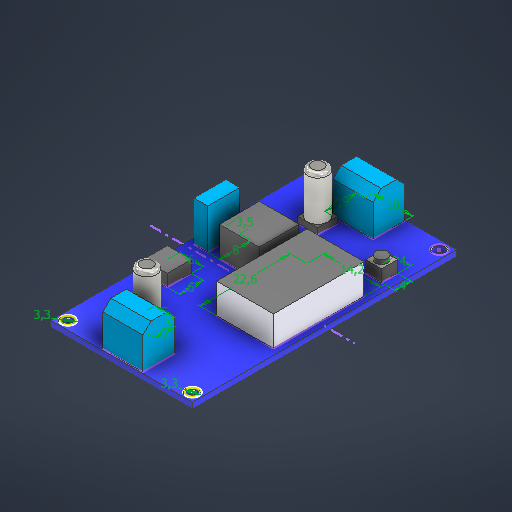
# Autodesk Inventor part: STEP_DOWN_LM2596
Saved by Autodesk Inventor 2027.1 (Build 311270010, 270A)
## iProperties
Created: 2026-08-16
Part Number: STEP_DOWN_LM2596
Material: Genérico
Document SubType Name: Modeling
Designer: Evellyn
Density: 1 g/cm^3
Appearance: Padrão
Author: Evellyn
Autodesk Inventor part; units mm, degrees
ref_plane "YZ Plane" through (0, 0, 0) normal (1, 0, 0) x (0, 1, 0)
ref_plane "XZ Plane" through (0, 0, 0) normal (0, 1, 0) x (-1, 0, 0)
ref_plane "XY Plane" through (0, 0, 0) normal (0, 0, 1) x (1, 0, 0)
sketch "Esboço1" plane through (0, 0, 0) normal (0, 1, 0) x (-1, 0, 0)
  line L0 (-17.7, -33) -> (17.7, -33)
  line L1 (17.7, -33) -> (17.7, 33)
  line L2 (17.7, 33) -> (-17.7, 33)
  line L3 (-17.7, 33) -> (-17.7, -33)
  line L4 (-17.7, -33) -> (17.7, 33) construction
  line L5 (17.7, -33) -> (-17.7, 33) construction
  circle A0 centre (15.55, 30.85) radius 1.35
  circle A1 centre (-15.55, 30.85) radius 1.35
  circle A2 centre (15.55, -30.85) radius 1.35
  circle A3 centre (-15.55, -30.85) radius 1.35
  point P0 (0, 0)
  dimension "d0" = 35.4
  dimension "d1" = 66
  dimension "d2" = 2.7
  dimension "d4" = 0.8
  dimension "d5" = 0.8
  dimension "d6" = 2.7
  dimension "d8" = 0.8
  dimension "d9" = 0.8
  constraints: 12 end point, 4 centre point, 2 midpoint, 2 parallel, 1 horizontal, 1 perpendicular
  measures "d0" distance of L2.end L1.end
  measures "d1" distance of L1.end L0.end
  measures "d2" diameter of A0
  measures "d4" distance edge to line of A0 L2
  measures "d5" distance edge to line of A0 L1
  measures "d6" diameter of A1
  measures "d8" distance edge to line of A1 L3
  measures "d9" distance edge to line of A1 L2
extrude "Extrusão1" add sketch "Esboço1" along normal blind 1.5
sketch "Esboço2" plane through (0, 1.5, 0) normal (0, 1, 0) x (1, 0, 0)
  line L0 (5, 24.7918) -> (-5, 24.7918)
  line L1 (-5, 24.7918) -> (-5, 32.6918)
  line L2 (-5, 32.6918) -> (5, 32.6918)
  line L3 (5, 32.6918) -> (5, 24.7918)
  line L4 (5, 24.7918) -> (-5, 32.6918) construction
  line L5 (-5, 24.7918) -> (5, 32.6918) construction
  line L6 (-26.0305, 0) -> (25.0606, 0)
  line L7 (5, -24.7918) -> (-5, -24.7918)
  line L8 (-5, -24.7918) -> (-5, -32.6918)
  line L9 (-5, -32.6918) -> (5, -32.6918)
  line L10 (5, -32.6918) -> (5, -24.7918)
  line L11 (16.2337, -11.3) -> (2.0337, -11.3)
  line L12 (2.0337, -11.3) -> (2.0337, 11.3)
  line L13 (2.0337, 11.3) -> (16.2337, 11.3)
  line L14 (16.2337, 11.3) -> (16.2337, -11.3)
  line L15 (16.2337, -11.3) -> (2.0337, 11.3) construction
  line L16 (2.0337, -11.3) -> (16.2337, 11.3) construction
  line L17 (-7.8666, -23.8534) -> (-2.8666, -23.8534)
  line L18 (-2.8666, -23.8534) -> (-2.8666, -18.8534)
  line L19 (-2.8666, -18.8534) -> (-7.8666, -18.8534)
  line L20 (-7.8666, -18.8534) -> (-7.8666, -23.8534)
  line L21 (-7.8666, 23.8534) -> (-2.8666, 23.8534)
  line L22 (-2.8666, 23.8534) -> (-2.8666, 18.8534)
  line L23 (-2.8666, 18.8534) -> (-7.8666, 18.8534)
  line L24 (-7.8666, 18.8534) -> (-7.8666, 23.8534)
  line L25 (11.4703, 16.4532) -> (15.4703, 16.4532)
  line L26 (15.4703, 16.4532) -> (15.4703, 20.4532)
  line L27 (15.4703, 20.4532) -> (11.4703, 20.4532)
  line L28 (11.4703, 20.4532) -> (11.4703, 16.4532)
  line L29 (-16.3029, 1.3386) -> (-12.8029, 1.3386)
  line L30 (-12.8029, 1.3386) -> (-12.8029, 9.3386)
  line L31 (-12.8029, 9.3386) -> (-16.3029, 9.3386)
  line L32 (-16.3029, 9.3386) -> (-16.3029, 1.3386)
  line L33 (-9.8893, 1.3386) -> (0, 1.3386)
  line L34 (0, 1.3386) -> (0, 11.3)
  line L35 (0, 11.3) -> (-9.8893, 11.3)
  line L36 (-9.8893, 11.3) -> (-9.8893, 1.3386)
  line L37 (-16.3029, -11.3) -> (-10.3029, -11.3)
  line L38 (-10.3029, -11.3) -> (-10.3029, -5.3)
  line L39 (-10.3029, -5.3) -> (-16.3029, -5.3)
  line L40 (-16.3029, -5.3) -> (-16.3029, -11.3)
  circle A0 centre (-15.55, -30.85) radius 1.35 projected
  circle A1 centre (-15.55, -30.85) radius 1.65
  circle A2 centre (15.55, -30.85) radius 1.35 projected
  circle A3 centre (15.55, -30.85) radius 1.65
  circle A4 centre (-15.55, 30.85) radius 1.65
  circle A5 centre (15.55, 30.85) radius 1.65
  point P0 (0, 0)
  point P1 (0, 28.7418)
  point P2 (0, -28.7418)
  point P3 (9.1337, 0)
  dimension "d12" = 10
  dimension "d13" = 7.9
  dimension "d14" = 14.2
  dimension "d15" = 22.6
  dimension "d16" = 5
  dimension "d17" = 5
  dimension "d18" = 4
  dimension "d19" = 4
  dimension "d20" = 3.5
  dimension "d21" = 8
  dimension "d22" = 6
  dimension "d23" = 6
  dimension "d42" = 3.3
  dimension "d43" = 3.3
  constraints: 82 end point, 14 parallel, 11 symmetric about line, 8 horizontal, 7 perpendicular, 4 centre point, 4 midpoint, 2 coincident, 2 point on line, 2 other
  measures "d12" distance of L1.end L2.end
  measures "d13" distance of L0.end L1.end
  measures "d14" distance of L12.end L13.end
  measures "d15" distance of L11.end L12.end
  measures "d16" distance of L19.end L18.end
  measures "d17" distance of L18.end L17.end
  measures "d18" distance of L27.end L26.end
  measures "d19" distance of L26.end L25.end
  measures "d20" distance of L31.end L30.end
  measures "d21" distance of L30.end L29.end
  measures "d22" distance of L39.end L38.end
  measures "d23" distance of L38.end L37.end
  measures "d42" diameter of A1
  measures "d43" diameter of A3
extrude "Extrusão2" add sketch "Esboço2" along normal blind 10 contours L0 L1 L2 L3 | L10 L9 L8 L7 | L32 L31 L30 L29
chamfer "Chanfro1" distance 2 angle 45 4 edges at (0, 11.5, -24.7918) (0, 11.5, -32.6918) (0, 11.5, 32.6918) (0, 11.5, 24.7918)
extrude "Extrusão3" add sketch "Esboço2" along normal blind 7.5 contours L12 L13 L14 L6 | L6 L14 L11 L12 | L36 L35 L34 L33
extrude "Extrusão4" add sketch "Esboço2" along normal blind 3 contours L28 L27 L26 L25 | L40 L39 L38 L37
extrude "Extrusão5" add sketch "Esboço2" along normal blind 1.5 contours L20 L19 L18 L17 | L21 L22 L23 L24
sketch "Esboço3" plane through (0, 3, 0) normal (0, 1, 0) x (1, 0, 0)
  line L0 (-7.8666, -18.8534) -> (-7.8666, -23.8534) projected
  line L1 (-7.8666, -23.8534) -> (-2.8666, -23.8534) projected
  line L2 (-2.8666, -18.8534) -> (-7.8666, -18.8534) projected
  line L3 (-2.8666, -23.8534) -> (-2.8666, -18.8534) projected
  circle A0 centre (-5.3666, -21.3534) radius 2.5
  point P0 (0, 0)
  constraints: 1 centre point
sketch "Esboço4" plane through (0, 3, 0) normal (0, 1, 0) x (1, 0, 0)
  line L0 (-7.8666, 23.8534) -> (-7.8666, 18.8534) projected
  line L1 (-7.8666, 18.8534) -> (-2.8666, 18.8534) projected
  line L2 (-2.8666, 23.8534) -> (-7.8666, 23.8534) projected
  line L3 (-2.8666, 18.8534) -> (-2.8666, 23.8534) projected
  circle A0 centre (-5.3666, 21.3534) radius 2.5
  point P0 (0, 0)
  constraints: 1 centre point
sketch "Esboço7" plane through (0, 4.5, 0) normal (0, 1, 0) x (1, 0, 0)
  line L0 (11.4703, 20.4532) -> (11.4703, 16.4532) projected
  line L1 (11.4703, 16.4532) -> (15.4703, 16.4532) projected
  line L2 (15.4703, 20.4532) -> (11.4703, 20.4532) projected
  line L3 (15.4703, 16.4532) -> (15.4703, 20.4532) projected
  circle A0 centre (13.4703, 18.4532) radius 1.5205
  point P0 (0, 0)
  constraints: 1 centre point
extrude "Extrusão6" add sketch "Esboço3" along normal blind 11 contours A0
extrude "Extrusão7" add sketch "Esboço4" along normal blind 11 contours A0
extrude "Extrusão8" add sketch "Esboço7" along normal blind 1 contours A0
fillet "Arredondamento1" radius 1 2 edges at (-7.8666, 14, 21.3534) (-7.8666, 14, -21.3534)
extrude "Extrusão9" cut sketch "Esboço2" against normal blind 0.1 contours A1 | A3 | A4 | A5
